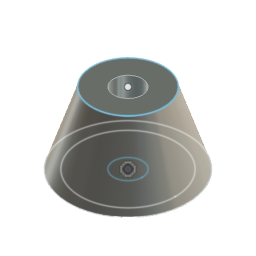
Mazda MX5 Ariel Adapter R1 (Autodesk Fusion 360 design; units mm, degrees)
Autodesk Fusion 360 part; units mm, degrees
sketch "Adapter" plane through (0, 0, 0) normal (0, 0, 1) x (1, 0, 0)
  circle A0 centre (0, 0) radius 12.5
  circle A1 through (7.5, 0, 15) (-3.75, 6.4952, 15) (-3.75, -6.4952, 15)
  circle A2 centre (0, 0) radius 3
  circle A3 centre (0, 0) radius 10
  dimension "d1" = 25
  dimension "d2" = 15
  dimension "d3" = 6
  dimension "d6" = 20
  constraint coincident A0.centre A2.centre
  measures "d1" diameter of A0
  measures "d3" diameter of A2
  measures "d6" diameter of A3
loft "Extrude Adapter" add profiles "Adapter", "Adapter" section 1 contours A0 | A3 section 2 contours A1 in plane through (0, 0, 15) normal (0, 0, 1)
extrude "Extrude Screw" cut sketch "Adapter" along normal blind 15 contours A2
extrude "Extrude Spacing" cut sketch "Adapter" along normal blind 3 contours A3
named bodies: "Adapter"
